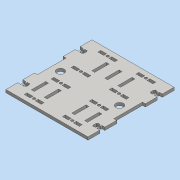
# Autodesk Inventor part: Y-Anchor_Back
Saved by Autodesk Inventor 2016 SP1 (Build 200210100, 210)
## iProperties
Created: 2015-12-01
Part Number: Y-Anchor_Back
Material: Generic
Document SubType Name: Modeling
Designer: Mohamed A.
Density: 1 g/cm^3
Appearance: Default
Author: Mohamed A.
Autodesk Inventor part; units mm, degrees
ref_plane "YZ Plane" through (0, 0, 0) normal (1, 0, 0) x (0, 1, 0)
ref_plane "XZ Plane" through (0, 0, 0) normal (0, 1, 0) x (-1, 0, 0)
ref_plane "XY Plane" through (0, 0, 0) normal (0, 0, 1) x (1, 0, 0)
sketch "Sketch1" plane through (0, 0, 0) normal (0, 0, 1) x (1, 0, 0)
  circle A0 centre (0, 0) radius 7.5
  circle A1 centre (18.5, 0) radius 2.25
  circle A2 centre (-18.5, 0) radius 2.25
  circle A3 centre (30.8333, 0) radius 3.9
  circle A4 centre (-30.8333, 0) radius 3.9
  line L0 (-51.1513, 0) -> (71.4472, 0) construction
  line L1 (15.8333, -16.9294) -> (39.8333, -16.9294) construction
  line L2 (39.8333, -16.9294) -> (39.8333, -31.9294) construction
  line L3 (39.8333, -31.9294) -> (15.8333, -31.9294) construction
  line L4 (15.8333, -31.9294) -> (15.8333, -16.9294) construction
  arc A5 (-21.25, 4.9867) -> (-24, 2.1319) centre (-18.93, 0) ccw construction
  line L5 (-24, -2.1319) -> (-24, 2.1319) construction
  arc A6 (-24, -2.1319) -> (-21.25, -4.9867) centre (-18.93, 0) ccw construction
  line L6 (-10.125, -8.9294) -> (-21.25, -4.9867) construction
  arc A7 (-10.125, -8.9294) -> (10.125, -8.9294) centre (0, 0) ccw construction
  line L7 (21.25, -4.9867) -> (10.125, -8.9294) construction
  arc A8 (21.25, -4.9867) -> (24, -2.1319) centre (18.93, 0) ccw construction
  line L8 (24, 2.1319) -> (24, -2.1319) construction
  arc A9 (24, 2.1319) -> (21.25, 4.9867) centre (18.93, 0) ccw construction
  line L9 (10.125, 8.9294) -> (21.25, 4.9867) construction
  arc A10 (10.125, 8.9294) -> (-10.125, 8.9294) centre (0, 0) ccw construction
  line L10 (-21.25, 4.9867) -> (-10.125, 8.9294) construction
  line L11 (0, 50.1847) -> (0, -53.8877) construction
  line L12 (11.0648, -8.9294) -> (17.2667, -8.9294)
  line L13 (28.7685, -8.9294) -> (28.7685, -11.9294)
  line L14 (28.7685, -11.9294) -> (22.5667, -11.9294)
  line L15 (11.0648, -11.9294) -> (11.0648, -8.9294)
  line L16 (27.8333, -15.5254) -> (27.8333, -35.4643) construction
  line L17 (48.9929, -24.4294) -> (9.7408, -24.4294) construction
  line L18 (19.9167, -5.8226) -> (19.9167, -14.0511) construction
  line L19 (64.5029, 29.9529) -> (40.2998, 29.9529) construction
  line L20 (34.8333, 31.4529) -> (34.8333, 28.4529)
  line L21 (35.4333, 32.6029) -> (37.8333, 32.6029)
  line L22 (37.8333, 27.3029) -> (35.4333, 27.3029)
  line L23 (39.8333, 32.6029) -> (42.8333, 32.6029)
  line L24 (42.8333, 27.3029) -> (39.8333, 27.3029)
  line L25 (39.8333, 27.3029) -> (39.8333, 28.4529)
  line L26 (42.8333, 14.9765) -> (42.8333, 27.3029)
  line L27 (42.8333, 32.6029) -> (42.8333, 44.9294)
  line L28 (39.8333, 31.4529) -> (37.8333, 31.4529)
  line L29 (35.4333, 31.4529) -> (34.8333, 31.4529)
  line L30 (34.8333, 28.4529) -> (35.4333, 28.4529)
  line L31 (37.8333, 28.4529) -> (39.8333, 28.4529)
  line L32 (37.8333, 32.6029) -> (37.8333, 31.4529)
  line L33 (37.8333, 28.4529) -> (37.8333, 27.3029)
  line L34 (35.4333, 27.3029) -> (35.4333, 28.4529)
  line L35 (35.4333, 31.4529) -> (35.4333, 32.6029)
  line L36 (39.8333, 32.6029) -> (39.8333, 31.4529)
  line L37 (39.8333, 28.4529) -> (39.8333, 27.3029)
  line L38 (39.8333, 31.4529) -> (39.8333, 32.6029)
  line L39 (42.8333, 14.9765) -> (39.8333, 14.9765)
  line L40 (39.8333, 14.9765) -> (39.8333, -14.9765)
  line L41 (39.8333, -14.9765) -> (42.8333, -14.9765)
  line L42 (34.8333, -31.4529) -> (34.8333, -28.4529)
  line L43 (35.4333, -32.6029) -> (37.8333, -32.6029)
  line L44 (37.8333, -27.3029) -> (35.4333, -27.3029)
  line L45 (39.8333, -32.6029) -> (42.8333, -32.6029)
  line L46 (42.8333, -27.3029) -> (39.8333, -27.3029)
  line L47 (39.8333, -27.3029) -> (39.8333, -28.4529)
  line L48 (42.8333, -14.9765) -> (42.8333, -27.3029)
  line L49 (42.8333, -32.6029) -> (42.8333, -44.9294)
  line L50 (39.8333, -31.4529) -> (37.8333, -31.4529)
  line L51 (35.4333, -31.4529) -> (34.8333, -31.4529)
  line L52 (34.8333, -28.4529) -> (35.4333, -28.4529)
  line L53 (37.8333, -28.4529) -> (39.8333, -28.4529)
  line L54 (37.8333, -32.6029) -> (37.8333, -31.4529)
  line L55 (37.8333, -28.4529) -> (37.8333, -27.3029)
  line L56 (35.4333, -27.3029) -> (35.4333, -28.4529)
  line L57 (35.4333, -31.4529) -> (35.4333, -32.6029)
  line L58 (39.8333, -32.6029) -> (39.8333, -31.4529)
  line L59 (-34.8333, 31.4529) -> (-34.8333, 28.4529)
  line L60 (-35.4333, 32.6029) -> (-37.8333, 32.6029)
  line L61 (-37.8333, 27.3029) -> (-35.4333, 27.3029)
  line L62 (-39.8333, 32.6029) -> (-42.8333, 32.6029)
  line L63 (-42.8333, 27.3029) -> (-39.8333, 27.3029)
  line L64 (-39.8333, 27.3029) -> (-39.8333, 28.4529)
  line L65 (-42.8333, 14.9765) -> (-42.8333, 27.3029)
  line L66 (-42.8333, 32.6029) -> (-42.8333, 44.9294)
  line L67 (-39.8333, 31.4529) -> (-37.8333, 31.4529)
  line L68 (-35.4333, 31.4529) -> (-34.8333, 31.4529)
  line L69 (-34.8333, 28.4529) -> (-35.4333, 28.4529)
  line L70 (-37.8333, 28.4529) -> (-39.8333, 28.4529)
  line L71 (-37.8333, 32.6029) -> (-37.8333, 31.4529)
  line L72 (-37.8333, 28.4529) -> (-37.8333, 27.3029)
  line L73 (-35.4333, 27.3029) -> (-35.4333, 28.4529)
  line L74 (-35.4333, 31.4529) -> (-35.4333, 32.6029)
  line L75 (-39.8333, 32.6029) -> (-39.8333, 31.4529)
  line L76 (-42.8333, 14.9765) -> (-39.8333, 14.9765)
  line L77 (-39.8333, 14.9765) -> (-39.8333, -14.9765)
  line L78 (-39.8333, -14.9765) -> (-42.8333, -14.9765)
  line L79 (-42.8333, -32.6029) -> (-42.8333, -44.9294)
  line L80 (-39.8333, -32.6029) -> (-42.8333, -32.6029)
  line L81 (-39.8333, -32.6029) -> (-39.8333, -31.4529)
  line L82 (-39.8333, -31.4529) -> (-37.8333, -31.4529)
  line L83 (-37.8333, -32.6029) -> (-37.8333, -31.4529)
  line L84 (-35.4333, -32.6029) -> (-37.8333, -32.6029)
  line L85 (-35.4333, -31.4529) -> (-35.4333, -32.6029)
  line L86 (-35.4333, -31.4529) -> (-34.8333, -31.4529)
  line L87 (-34.8333, -31.4529) -> (-34.8333, -28.4529)
  line L88 (-34.8333, -28.4529) -> (-35.4333, -28.4529)
  line L89 (-35.4333, -27.3029) -> (-35.4333, -28.4529)
  line L90 (-37.8333, -27.3029) -> (-35.4333, -27.3029)
  line L91 (-37.8333, -28.4529) -> (-37.8333, -27.3029)
  line L92 (-37.8333, -28.4529) -> (-39.8333, -28.4529)
  line L93 (-39.8333, -27.3029) -> (-39.8333, -28.4529)
  line L94 (-42.8333, -27.3029) -> (-39.8333, -27.3029)
  line L95 (-42.8333, -14.9765) -> (-42.8333, -27.3029)
  line L96 (-42.8333, 44.9294) -> (42.8333, 44.9294)
  line L97 (42.8333, -44.9294) -> (-42.8333, -44.9294)
  line L98 (10.125, -8.9294) -> (-10.125, -8.9294) construction
  line L99 (22.5667, -8.9294) -> (22.5667, -11.9294)
  line L100 (17.2667, -8.9294) -> (17.2667, -11.9294)
  line L101 (22.5667, -8.9294) -> (28.7685, -8.9294)
  line L102 (17.2667, -11.9294) -> (11.0648, -11.9294)
  circle A11 centre (19.9167, -10.4294) radius 1.4
  line L103 (11.0648, -39.9294) -> (17.2667, -39.9294)
  line L104 (28.7685, -39.9294) -> (28.7685, -36.9294)
  line L105 (28.7685, -36.9294) -> (22.5667, -36.9294)
  line L106 (11.0648, -36.9294) -> (11.0648, -39.9294)
  line L107 (22.5667, -39.9294) -> (22.5667, -36.9294)
  line L108 (17.2667, -39.9294) -> (17.2667, -36.9294)
  line L109 (22.5667, -39.9294) -> (28.7685, -39.9294)
  line L110 (17.2667, -36.9294) -> (11.0648, -36.9294)
  circle A12 centre (19.9167, -38.4294) radius 1.4
  line L111 (26.3333, -16.9294) -> (29.3333, -16.9294)
  line L112 (29.3333, -16.9294) -> (29.3333, -31.9294)
  line L113 (29.3333, -31.9294) -> (26.3333, -31.9294)
  line L114 (26.3333, -31.9294) -> (26.3333, -16.9294)
  line L115 (15.8333, -16.9294) -> (12.8333, -16.9294)
  line L116 (12.8333, -16.9294) -> (12.8333, -31.9294)
  line L117 (12.8333, -31.9294) -> (15.8333, -31.9294)
  line L118 (15.8333, -31.9294) -> (15.8333, -16.9294)
  line L119 (-11.0648, -8.9294) -> (-17.2667, -8.9294)
  line L120 (-28.7685, -8.9294) -> (-28.7685, -11.9294)
  line L121 (-28.7685, -11.9294) -> (-22.5667, -11.9294)
  line L122 (-11.0648, -11.9294) -> (-11.0648, -8.9294)
  line L123 (-22.5667, -8.9294) -> (-22.5667, -11.9294)
  line L124 (-17.2667, -8.9294) -> (-17.2667, -11.9294)
  line L125 (-22.5667, -8.9294) -> (-28.7685, -8.9294)
  line L126 (-17.2667, -11.9294) -> (-11.0648, -11.9294)
  circle A13 centre (-19.9167, -10.4294) radius 1.4
  circle A14 centre (-19.9167, -38.4294) radius 1.4
  line L127 (-22.5667, -39.9294) -> (-28.7685, -39.9294)
  line L128 (-22.5667, -39.9294) -> (-22.5667, -36.9294)
  line L129 (-28.7685, -36.9294) -> (-22.5667, -36.9294)
  line L130 (-28.7685, -39.9294) -> (-28.7685, -36.9294)
  line L131 (-11.0648, -39.9294) -> (-17.2667, -39.9294)
  line L132 (-17.2667, -39.9294) -> (-17.2667, -36.9294)
  line L133 (-17.2667, -36.9294) -> (-11.0648, -36.9294)
  line L134 (-11.0648, -36.9294) -> (-11.0648, -39.9294)
  line L135 (-26.3333, -16.9294) -> (-29.3333, -16.9294)
  line L136 (-29.3333, -16.9294) -> (-29.3333, -31.9294)
  line L137 (-29.3333, -31.9294) -> (-26.3333, -31.9294)
  line L138 (-26.3333, -31.9294) -> (-26.3333, -16.9294)
  line L139 (-15.8333, -16.9294) -> (-12.8333, -16.9294)
  line L140 (-12.8333, -16.9294) -> (-12.8333, -31.9294)
  line L141 (-12.8333, -31.9294) -> (-15.8333, -31.9294)
  line L142 (-15.8333, -31.9294) -> (-15.8333, -16.9294)
  line L143 (11.0648, 8.9294) -> (17.2667, 8.9294)
  line L144 (28.7685, 8.9294) -> (28.7685, 11.9294)
  line L145 (28.7685, 11.9294) -> (22.5667, 11.9294)
  line L146 (11.0648, 11.9294) -> (11.0648, 8.9294)
  line L147 (22.5667, 8.9294) -> (22.5667, 11.9294)
  line L148 (17.2667, 8.9294) -> (17.2667, 11.9294)
  line L149 (22.5667, 8.9294) -> (28.7685, 8.9294)
  line L150 (17.2667, 11.9294) -> (11.0648, 11.9294)
  circle A15 centre (19.9167, 10.4294) radius 1.4
  circle A16 centre (19.9167, 38.4294) radius 1.4
  line L151 (22.5667, 39.9294) -> (28.7685, 39.9294)
  line L152 (22.5667, 39.9294) -> (22.5667, 36.9294)
  line L153 (28.7685, 36.9294) -> (22.5667, 36.9294)
  line L154 (28.7685, 39.9294) -> (28.7685, 36.9294)
  line L155 (11.0648, 39.9294) -> (17.2667, 39.9294)
  line L156 (17.2667, 39.9294) -> (17.2667, 36.9294)
  line L157 (17.2667, 36.9294) -> (11.0648, 36.9294)
  line L158 (11.0648, 36.9294) -> (11.0648, 39.9294)
  line L159 (-28.7685, 11.9294) -> (-22.5667, 11.9294)
  line L160 (-28.7685, 8.9294) -> (-28.7685, 11.9294)
  line L161 (-22.5667, 8.9294) -> (-28.7685, 8.9294)
  line L162 (-22.5667, 8.9294) -> (-22.5667, 11.9294)
  circle A17 centre (-19.9167, 10.4294) radius 1.4
  line L163 (-17.2667, 8.9294) -> (-17.2667, 11.9294)
  line L164 (-11.0648, 8.9294) -> (-17.2667, 8.9294)
  line L165 (-11.0648, 11.9294) -> (-11.0648, 8.9294)
  line L166 (-17.2667, 11.9294) -> (-11.0648, 11.9294)
  line L167 (-17.2667, 36.9294) -> (-11.0648, 36.9294)
  line L168 (-11.0648, 36.9294) -> (-11.0648, 39.9294)
  line L169 (-11.0648, 39.9294) -> (-17.2667, 39.9294)
  line L170 (-17.2667, 39.9294) -> (-17.2667, 36.9294)
  circle A18 centre (-19.9167, 38.4294) radius 1.4
  line L171 (-22.5667, 39.9294) -> (-22.5667, 36.9294)
  line L172 (-22.5667, 39.9294) -> (-28.7685, 39.9294)
  line L173 (-28.7685, 39.9294) -> (-28.7685, 36.9294)
  line L174 (-28.7685, 36.9294) -> (-22.5667, 36.9294)
  line L175 (12, 31.9294) -> (-12, 31.9294) construction
  line L176 (-12, 31.9294) -> (-12, 16.9294) construction
  line L177 (-12, 16.9294) -> (12, 16.9294) construction
  line L178 (12, 16.9294) -> (12, 31.9294) construction
  line L179 (-17.778, 24.4294) -> (21.8712, 24.4294) construction
  line L180 (12, 31.9294) -> (15, 31.9294)
  line L181 (15, 31.9294) -> (15, 16.9294)
  line L182 (15, 16.9294) -> (12, 16.9294)
  line L183 (12, 16.9294) -> (12, 31.9294)
  line L184 (-12, 31.9294) -> (-15, 31.9294)
  line L185 (-15, 31.9294) -> (-15, 16.9294)
  line L186 (-15, 16.9294) -> (-12, 16.9294)
  line L187 (-12, 16.9294) -> (-12, 31.9294)
  line L188 (-1.5, 16.9294) -> (1.5, 16.9294)
  line L189 (1.5, 16.9294) -> (1.5, 31.9294)
  line L190 (1.5, 31.9294) -> (-1.5, 31.9294)
  line L191 (-1.5, 31.9294) -> (-1.5, 16.9294)
  point P0 (0, 0)
  point P1 (22.8911, -3.8157)
  dimension "d2" = 4.5
  dimension "d3" = 4.5
  dimension "d4" = 7.8
  dimension "d5" = 7.8
  dimension "d61" = 15
  dimension "d62" = 24
  dimension "d63" = 15
  dimension "d64" = 3
  dimension "d76" = 2.4
  dimension "d79" = 3
  dimension "d81" = 29.9529
  dimension "d82" = 8
  dimension "d83" = 5
  dimension "d84" = 3
  dimension "d85" = 29.9529
  dimension "d87" = 17.7037
  dimension "d88" = 39.8333
  dimension "d89" = 12
  dimension "d90" = 5
  dimension "d92" = 5.3
  dimension "d93" = 2.8
  dimension "d94" = 5
  dimension "d95" = 3
  dimension "d96" = 3
  dimension "d97" = 24
  dimension "d98" = 15
  dimension "d99" = 3
  dimension "d100" = 3
  dimension "d101" = 3
  constraints: 384 end point, 129 symmetric about line, 34 parallel, 20 horizontal, 19 centre point, 19 perpendicular, 15 collinear, 13 point on circle, 10 point on line, 6 vertical, 36 other
  measures "d2" diameter of A1
  measures "d3" diameter of A2
  measures "d4" diameter of A3
  measures "d5" diameter of A4
  measures "d61" diameter of A0
  measures "d62" distance of L2.end L3.end
  measures "d63" distance between parallel lines of L3 L1
  measures "d64" distance of L13.start L13.end
  measures "d76" distance of L22.start L22.end
  measures "d79" distance of L26.start L39.end
  measures "d81" distance of L27.end L26.start
  measures "d82" distance between parallel lines of L26 L20
  measures "d83" distance between parallel lines of L27 L32
  measures "d84" distance between parallel lines of L27 L36
  measures "d85" distance between parallel lines of L41 L39
  measures "d87" distance between parallel lines of L15 L13
  measures "d88" distance between parallel lines of L40 L11
  measures "d89" distance from line of L26 A3.centre
  measures "d90" distance between parallel lines of L1 L14
  measures "d92" distance between parallel lines of L100 L99
  measures "d93" diameter of A11
  measures "d94" distance between parallel lines of L97 L109
  measures "d95" distance of L112.end L113.end
  measures "d96" distance of L117.end L116.end
  measures "d97" distance of L177.end L176.end
  measures "d98" distance of L176.end L175.end
  measures "d99" distance of L181.end L182.end
  measures "d100" distance of L186.end L185.end
  measures "d101" distance of L190.end L189.end
extrude "Extrusion1" add sketch "Sketch1" against normal blind 3 contours A0 | A1 | A2 | L20 L30 L34 L22 L33 L31 L25 L24 L26 L39 L40 L41 L48 L46 L47 L53 L55 L44 L56 L52 L42 L51 L57 L43 L54 L50 L58 L45 L49 L97 L79 L80 L81 L82 L83 L84 L85 L86 L87 L88 L89 L90 L91 L92 L93 L94 L95 L78 L77 L76 L65 L63 L64 L70 L72 L61 L73 L69 L59 L68 L74 L60 L71 L67 L75 L62 L66 L96 L27 L23 L36 L28 L32 L21 L35 L29
body "Solid1"
